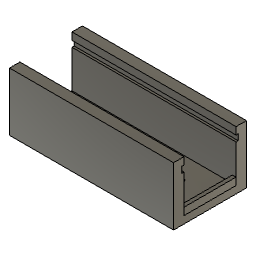
ST-Link Holder v3 (Autodesk Fusion 360 design; units mm, degrees)
Autodesk Fusion 360 part; units mm, degrees
sketch "Main Body" plane through (0, 0, 0) normal (1, 0, 0) x (0, 1, 0)
  line L0 (7.15, 16) -> (10, 16)
  line L1 (10, 16) -> (10, 0)
  line L2 (10, 0) -> (0, 0)
  line L3 (7.15, 16) -> (7.15, 14)
  line L4 (7.15, 14) -> (7.75, 14)
  line L5 (7.75, 14) -> (7.75, 12.35)
  line L6 (7.75, 12.35) -> (7.15, 12.35)
  line L7 (7.15, 12.35) -> (7.15, 2)
  line L8 (7.15, 2) -> (0, 2)
  line L9 (0, 16.5) -> (0, -3.5) construction
  line L10 (-10, 16) -> (-10, 0)
  line L11 (-7.15, 14) -> (-7.75, 14)
  line L12 (-7.75, 12.35) -> (-7.15, 12.35)
  line L13 (-10, 0) -> (0, 0)
  line L14 (-7.15, 12.35) -> (-7.15, 2)
  line L15 (-7.75, 14) -> (-7.75, 12.35)
  line L16 (-7.15, 2) -> (0, 2)
  line L17 (-7.15, 16) -> (-7.15, 14)
  line L18 (-7.15, 16) -> (-10, 16)
  point P0 (0, 16.5)
  point P1 (0, -3.5)
  dimension "d1" = 14
  dimension "d3" = 7.75
  dimension "d4" = 2
  dimension "d5" = 0.6
  dimension "d6" = 0.6
  dimension "d7" = 1.65
  dimension "d25" = 10
  dimension "d26" = 2
  constraint horizontal L0
  constraint perpendicular L0 L1
  constraint coincident L2.end L13.end
  constraint perpendicular L1 L2
  constraint perpendicular L0 L3
  constraint perpendicular L3 L4
  constraint perpendicular L4 L5
  constraint perpendicular L3 L6
  constraint perpendicular L6 L7
  constraint perpendicular L7 L8
  constraint vertical L9
  constraint coincident L8.end L9
  constraint symmetric L2.end L9 L13.end
  constraint symmetric L0.start L9 L17.start
  constraint symmetric L0.end L9 L10.start
  constraint symmetric L1.end L9 L10.end
  constraint symmetric L3.end L9 L11.start
  constraint symmetric L4.end L9 L11.end
  constraint symmetric L5.end L9 L12.start
  constraint symmetric L6.end L9 L12.end
  constraint symmetric L7.end L9 L14.end
  constraint symmetric L8.end L9 L16.end
  constraint symmetric P0 L9 L9.start
  constraint symmetric P1 L9 L9.end
  measures "d1" distance of L2 L4
  measures "d3" distance of L5 L9
  measures "d4" distance of L0.start L3.end
  measures "d5" distance of L5.end L6.end
  measures "d6" distance of L3.end L4.end
  measures "d7" distance of L4.end L5.end
  measures "d25" distance of L1.end L2.end
  measures "d26" distance of L2 L8
extrude "Extrude1" add sketch "Main Body" along normal blind 45 makes body 1
sketch "Mounting Hole" plane through (0, 0, 0) normal (0, 0, -1) x (1, 0, 0)
  line L0 (0, 10) -> (0, -10)
  line L1 (0, -10) -> (45, -10)
  line L2 (45, -10) -> (45, 10)
  line L3 (45, 10) -> (0, 10)
  line L4 (0, -10) -> (45, 10) construction
  line L5 (45, -10) -> (0, 10) construction
  circle A0 centre (22.5, 0) radius 2
  dimension "d10" = 4
  constraint coincident L0.end L1.start
  constraint coincident L2.end L3.start
  constraint coincident L1.end L2.start
  constraint coincident L0.start L3.end
  constraint midpoint L4 A0.centre
  measures "d10" diameter of A0
extrude "Extrude2" cut sketch "Mounting Hole" against normal up to surface (2 mm away) contours A0 bodies 1
sketch "Sketch7" plane through (45, 0, 0) normal (1, 0, 0) x (0, 1, 0)
  line L0 (-7.15, 14) -> (-7.15, 16)
  line L1 (-7.15, 16) -> (-10, 16)
  line L2 (-10, 16) -> (-10, 0)
  line L3 (-10, 0) -> (10, 0)
  line L4 (10, 0) -> (10, 16)
  line L5 (10, 16) -> (7.15, 16)
  line L6 (7.15, 16) -> (7.15, 14)
  line L7 (7.15, 14) -> (7.75, 14)
  line L8 (7.75, 14) -> (7.75, 12.35)
  line L9 (7.75, 12.35) -> (7.15, 12.35)
  line L10 (7.15, 12.35) -> (7.15, 2)
  line L11 (7.15, 2) -> (-7.15, 2)
  line L12 (-7.15, 2) -> (-7.15, 12.35)
  line L13 (-7.15, 12.35) -> (-7.75, 12.35)
  line L14 (-7.75, 12.35) -> (-7.75, 14)
  line L15 (-7.75, 14) -> (-7.15, 14)
  line L16 (-7.15, 2) -> (7.15, 2)
  line L17 (7.15, 2) -> (7.15, 4)
  line L18 (7.15, 4) -> (-7.15, 4)
  line L19 (-7.15, 4) -> (-7.15, 2)
  dimension "d29" = 2
  constraint horizontal L16
  constraint vertical L17
  constraint horizontal L18
  constraint vertical L19
  constraint coincident L10 L17.end
  constraint coincident L11.end L12.start
  measures "d29" distance of L16 L18
extrude "Extrude5" add sketch "Sketch7" against normal blind 1 separate body contours L10 L11 L12 L16 L17 L18 L19 makes body 2
pattern_linear "R-Pattern2" count 3 spacing 12.75 along (1, 0, 0) both ways of "Extrude2"
equation "d6 = d5"
equation "d8 = HolderLength"
equation "HolderLength = LargeHolder"
equation "SmallHolder = 23 mm"
equation "LargeHolder = 45 mm"
